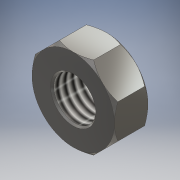
# Autodesk Inventor part: 2.5mm hex nut
Saved by Autodesk Inventor 2016 (Build 200138000, 138)
## iProperties
Created: 2016-07-05
Part Number: 2.5mm hex nut
Material: Steel, High Strength, Low Alloy
Document SubType Name: Modeling
Designer: Jonathan
Density: 7.85 g/cm^3
Appearance: Steel - Polished
Author: Jonathan
Autodesk Inventor part; units mm, degrees
ref_plane "YZ Plane" through (0, 0, 0) normal (1, 0, 0) x (0, 1, 0)
ref_plane "XZ Plane" through (0, 0, 0) normal (0, 1, 0) x (-1, 0, 0)
sketch "Sketch1" plane through (0, 0, 0) normal (0, 1, 0) x (-1, 0, 0)
  line L0 (2.45, 1.0148) -> (2.45, -1.0148)
  line L1 (2.45, -1.0148) -> (1.0148, -2.45)
  line L2 (1.0148, -2.45) -> (-1.0148, -2.45)
  line L3 (-1.0148, -2.45) -> (-2.45, -1.0148)
  line L4 (-2.45, -1.0148) -> (-2.45, 1.0148)
  line L5 (-2.45, 1.0148) -> (-1.0148, 2.45)
  line L6 (-1.0148, 2.45) -> (1.0148, 2.45)
  line L7 (1.0148, 2.45) -> (2.45, 1.0148)
  circle A0 centre (0, 0) radius 1.25
  point P0 (2.45, 0)
  point P1 (0, -2.45)
  dimension "d0" = 135
  dimension "d1" = 4.9
  dimension "d4" = 2.5
  constraints: 16 end point, 7 equal length, 2 midpoint, 2 parallel, 2 perpendicular, 1 centre point, 1 coincident, 1 horizontal alignment, 1 vertical, 1 vertical alignment
  measures "d0" angle of L7 L0
  measures "d1" distance between parallel lines of L4 L0
  measures "d4" diameter of A0
extrude "Extrusion1" add sketch "Sketch1" along normal mid plane 2
thread "Thread1" size "M2.5x0.45" class "6H" standard "ANSI Metric M Profile" full length
ref_plane "Work Plane1" through (1.0148, -1, 2.45) normal (0.9239, 0, -0.3827) x (-0.3827, 0, -0.9239)
sketch "Sketch3" plane through (1.0148, -1, 2.45) normal (0.9239, 0, -0.3827) x (-0.3827, 0, -0.9239)
  line L0 (0, 0) -> (0.7767, 0) projected
  line L1 (0, 2) -> (0, 0) projected
  line L2 (2.6519, -0.4) -> (2.6519, 2.4) projected
  line L3 (0, 0.2051) -> (0.2051, 0)
  line L4 (0.7767, 0) -> (0, 0) projected
  point P0 (2.6519, 1)
  dimension "d10" = 45
  dimension "d11" = 0.29
  constraints: 2 end point, 2 point on line
  measures "d10" angle of L1 L3
  measures "d11" distance of L3.start L3.end
revolve "Revolution1" cut sketch "Sketch3" angle 360 about axis through (0, -10, 0) along (0, 1, 0)
mirror "Mirror1" about plane through (0, 0, 0) normal (0, 1, 0) of "Revolution1"
chamfer "Chamfer1" distance 0.1 angle 45 1 edges at (1.25, -1, 0)
chamfer "Chamfer2" distance 0.1 angle 45 1 edges at (1.25, 1, 0)
body "Solid1"
